car pillar v9 (Autodesk Fusion 360 design; units mm, degrees)
Autodesk Fusion 360 part; units mm, degrees
note: some values were not read from the file. Chosen so that the rebuilt part matches the saved one: which bodies a step acts on; which face or edge a step refers to; the layout of a text. Set by a fixed rule: which sketch regions a step uses.
sketch "Sketch1" plane through (0, 0, 0) normal (0, 1, 0) x (1, 0, 0)
  line L0 (0, 0) -> (75, 0)
  line L1 (75, 0) -> (1014.8, 0)
  line L2 (1014.8, 0) -> (1014.8, -406)
  line L3 (1014.8, -406) -> (913.8, -406)
  arc A0 (75, 0) -> (913.8, -406) centre (913.8, 663.4845) ccw
  line L4 (1014.8, -406) -> (1014.8, -481)
  line L5 (1014.8, -481) -> (913.8, -481)
  arc A1 (0, 0) -> (913.8, -481) centre (913.8, 627.515) ccw
  dimension "d1" = 75
  dimension "d2" = 939.8
  dimension "d3" = 406
  dimension "d4" = 101
  dimension "d5" = 75
  dimension "d6" = 101
  constraint coincident L0.start A1.start
  constraint horizontal L0
  constraint parallel L0 L1
  constraint perpendicular L1 L2
  constraint perpendicular L2 L3
  constraint tangent L3 A0
  constraint perpendicular L3 L4
  constraint perpendicular L4 L5
  constraint tangent L5 A1
  measures "d1" distance of L0.start L0.end
  measures "d2" distance of L0.end L1.end
  measures "d3" distance of L1.end L2.end
  measures "d4" distance of L2.end L3.end
  measures "d5" distance of L2.end L4.end
  measures "d6" distance of L4.end L5.end
extrude "Extrude1" add sketch "Sketch1" along normal blind 76.2 contours L0 L3 A0 L4 L5 A1 makes body 1
sketch "Sketch2" plane through (0, 0, 0) normal (0, -1, 0) x (1, 0, 0)
  line L0 (0, 0) -> (75, 0)
  arc A0 (913.8, 406) -> (75, 0) centre (913.8, -663.4845) ccw
  line L1 (913.8, 406) -> (1014.8, 406)
  line L2 (1014.8, 406) -> (1014.8, 481)
  line L3 (1014.8, 481) -> (913.8, 481)
  arc A1 (913.8, 481) -> (0, 0) centre (913.8, -627.515) ccw
  line L4 (75, 0, -76.2) -> (0, 0, -76.2)
  arc A2 through (913.8, 481, -76.2) (397.4688, 353.4068, -76.2) (0, 0, -76.2)
  line L5 (913.8, 481, -76.2) -> (1014.8, 481, -76.2)
  line L6 (1014.8, 481, -76.2) -> (1014.8, 406, -76.2)
  line L7 (1014.8, 406, -76.2) -> (913.8, 406, -76.2)
  arc A3 through (913.8, 406, -76.2) (447.8543, 299.1638, -76.2) (75, 0, -76.2)
  arc A4 (913.8, 406) -> (75, 0) centre (913.8, -663.4845) ccw
  line L8 (178.7478, 202.2463) -> (217.2163, 148.0376)
  line L9 (317.7078, 307.0863) -> (348.9045, 244.64)
  line L10 (466.2211, 386.6244) -> (489.3869, 318.1827)
  line L11 (629.2604, 443.8592) -> (639.0355, 370.1022)
  line L12 (787.0542, 473.7302) -> (796.8801, 399.5897)
  line L13 (99.0687, 124.162) -> (134.4845, 68.9528)
  line L14 (913.8, 481) -> (913.8, 406)
  constraint coincident A1 L8.start
  constraint coincident A0 L8.end
  constraint coincident A1 L9.start
  constraint coincident A4 L9.end
  constraint coincident A1 L10.start
  constraint coincident A0 L10.end
  constraint coincident A1 L11.start
  constraint coincident A4 L11.end
  constraint coincident A1 L12.start
  constraint coincident A4 L12.end
  constraint parallel L11 L12
  constraint coincident A1 L13.start
  constraint coincident A0 L13.end
  constraint coincident L3.end A1.start
  constraint coincident A0.start L1.start
split "Split1" by curves path "Sketch2" along L8 bodies 1 makes body 2 at (156.5161, 50.8, 182.0074)
split "Split2" by curves path "Sketch2" along L13 bodies 2 makes body 3 at (20.4596, 25.4, 28.7993)
split "Split3" by curves path "Sketch2" along L9 L11 L12 L10 L14 bodies 1 makes body 4 at (301.4758, 50.8, 296.5329) makes body 5 at (333.5896, 50.8, 317.028) makes body 6 at (981.1333, 25.4, 406) makes body 7 at (555.7045, 50.8, 421.567) makes body 8 at (769.3289, 50.8, 471.5453)
fillet "Fillet1" radius 37.5 22 edges at (855.2522, 0, 404.3962) (964.3, 0, 406) (964.3, 76.2, 406) (855.2522, 76.2, 404.3962) (417.7808, 76.2, 284.0186) (281.2137, 76.2, 198.8563) (717.4036, 76.2, 387.8126) (563.2486, 76.2, 346.9168) (104.008, 76.2, 35.1098) (174.7917, 76.2, 109.6027) (174.7917, 0, 109.6027) (174.7917, 76.2, 109.6027) (104.008, 0, 35.1098) (104.008, 76.2, 35.1098) (563.2486, 0, 346.9168) (563.2486, 76.2, 346.9168) (717.4036, 0, 387.8126) (717.4036, 76.2, 387.8126) (281.2137, 0, 198.8563) (281.2137, 76.2, 198.8563) (417.7808, 0, 284.0186) (417.7808, 76.2, 284.0186) on bodies 1 2 3 4 5 6 7 8
shell "Shell2" thickness 3.5 removed faces 1 at (769.3289, 50.8, 471.5453) on bodies 8
shell "Shell3" thickness 3.5 removed faces 1 at (555.7045, 50.8, 421.567) on bodies 7
shell "Shell4" thickness 3.5 removed faces 1 at (333.5896, 50.8, 317.028) on bodies 5
shell "Shell5" thickness 3.5 removed faces 1 at (301.4758, 50.8, 296.5329) on bodies 4
shell "Shell6" thickness 3.5 removed faces 1 at (142.3659, 50.8, 168.5346) on bodies 2
shell "Shell7" thickness 3.5 removed faces 1 at (20.4596, 25.4, 28.7993) on bodies 3
shell "Shell8" thickness 3.5 removed faces 1 at (885.5756, 50.8, 480.6406) on bodies 1
shell "Shell9" thickness 3.5 removed faces 1 at (947.4667, 50.8, 481) on bodies 6
sketch "Sketch3" plane through (1014.8, 0, 0) normal (1, 0, 0) x (0, 1, 0)
  arc A0 (38.7, 406) -> (76.2, 443.5) centre (38.7, 443.5) ccw
  line L0 (76.2, 443.5) -> (76.2, 481)
  line L1 (76.2, 481) -> (0, 481)
  line L2 (0, 481) -> (0, 443.5)
  arc A1 (0, 443.5) -> (37.5, 406) centre (37.5, 443.5) ccw
  line L3 (37.5, 406) -> (38.7, 406)
  line L4 (38.1, 473.1824) -> (38.1, 422.3824)
  circle A2 centre (38.1, 427.3824) radius 5
  circle A3 centre (38.1, 468.1824) radius 5
  dimension "d21" = 38.1
  dimension "d22" = 50.8
  dimension "d23" = 7.8176
  dimension "d24" = 10
  dimension "d25" = 10
  constraint vertical L4
  constraint coincident L4.end A2
  constraint coincident L4.start A3
  measures "d21" distance of L2 L4
  measures "d22" distance of L4.start L4.end
  measures "d23" distance of L1 L4.start
  measures "d24" diameter of A2
  measures "d25" diameter of A3
extrude "Extrude2" cut sketch "Sketch3" against normal blind 10 contours L4 A3 | L4 A3 | L4 A2 | L4 A2 bodies 6
sketch "Sketch4" plane through (917.3, 0, 0) normal (1, 0, 0) x (0, 1, 0)
  arc A0 (38.7, 409.5) -> (72.7, 443.5) centre (38.7, 443.5) ccw
  line L0 (72.7, 443.5) -> (72.7, 481)
  line L1 (72.7, 481) -> (3.5, 481)
  line L2 (3.5, 481) -> (3.5, 443.5)
  arc A1 (3.5, 443.5) -> (37.5, 409.5) centre (37.5, 443.5) ccw
  line L3 (37.5, 409.5) -> (38.7, 409.5)
  line L4 (3.5, 481) -> (72.7, 481)
  line L5 (38.1, 481) -> (38.1, 430.2)
  line L6 (38.1, 481) -> (38.1, 468.3)
  line L7 (38.1, 430.2) -> (58.1, 430.2)
  line L8 (38.1, 430.2) -> (18.1, 430.2)
  circle A2 centre (18.1, 430.2) radius 1.575
  circle A3 centre (58.1, 430.2) radius 1.575
  circle A4 centre (38.1, 468.3) radius 1.575
  line L9 (33.6, 450.6777) -> (42.6, 450.6777) construction
  line L10 (42.6, 450.6777) -> (42.6, 461) construction
  line L11 (42.6, 461) -> (33.6, 461) construction
  line L12 (33.6, 461) -> (33.6, 450.6777) construction
  dimension "d28" = 90
  dimension "d29" = 50.8
  dimension "d30" = 12.7
  dimension "d31" = 20
  dimension "d32" = 20
  dimension "d33" = 3.15
  dimension "d34" = 3.15
  dimension "d35" = 3.15
  dimension "d102" = 15
  dimension "d103" = 20
  dimension "d104" = 9
  dimension "d105" = 30.1
  text T0 "7" font "Arial" height 15 bold align centre top in box 9 x 10.3223 at (33.6, 450.6777) x (1, 0) y (0, 1) spacing 1 by line height
  constraint coincident L1.end L2.start
  constraint coincident L0.end L1.start
  constraint midpoint L4 L5.start
  constraint perpendicular L4 L6
  constraint perpendicular L5 L7
  constraint horizontal L8
  constraint coincident L8.end A2.centre
  constraint coincident L7.end A3.centre
  constraint coincident L6.end A4.centre
  measures "d28" angle of L4 L5
  measures "d29" distance of L5.start L5.end
  measures "d30" distance of L5.start L6.end
  measures "d31" distance of L5.end L7.end
  measures "d32" distance of L5.end L8.end
  measures "d33" diameter of A2
  measures "d34" diameter of A3
  measures "d35" diameter of A4
  measures "d104" distance of L10
  measures "d105" distance of L2 L12
extrude "Extrude11" cut sketch "Sketch4" against normal blind 1.5 text T0 bodies 6
extrude "Extrude3" cut sketch "Sketch4" against normal blind 16 contours L5 L6 A4 | L5 L6 A4 | A2 | A3 bodies 1 6
sketch "Sketch6" plane through (838.6384, 0, 111.1453) normal (0.991332, 0, 0.131382) x (0, 1, 0)
  spline S0 degree 3 poles (38.7, 294.8481) (40.7978, 294.8481) (43.0889, 295.0551) (47.5758, 295.9478) (49.7717, 296.6335) (53.6482, 298.2395) (55.6859, 299.3078) (59.4901, 301.8503) (61.2567, 303.3244) (64.2239, 306.2922) (65.6979, 308.0594) (68.2402, 311.8649) (69.3084, 313.9032) (70.9144, 317.7812) (71.6002, 319.9783) (72.493, 324.4676) (72.7, 326.7598) (72.7, 328.8587) knots 10.072074 10.072074 10.072074 10.072074 10.70142 10.70142 11.330765 11.330765 11.960214 11.960214 12.589663 12.589663 13.219234 13.219234 13.848804 13.848804 14.478468 14.478468 15.108132 15.108132 15.108132 15.108132
  line L0 (72.7, 328.8587) -> (72.7, 366.1536)
  line L1 (72.7, 366.1536) -> (3.5, 366.1536)
  line L2 (3.5, 366.1536) -> (3.5, 328.8587)
  spline S1 degree 3 poles (3.5, 328.8587) (3.5, 326.7598) (3.707, 324.4676) (4.5998, 319.9783) (5.2856, 317.7812) (6.8916, 313.9032) (7.9598, 311.8649) (10.5021, 308.0594) (11.9761, 306.2922) (14.9433, 303.3244) (16.7099, 301.8503) (20.5141, 299.3078) (22.5518, 298.2395) (26.4283, 296.6335) (28.6242, 295.9478) (33.1111, 295.0551) (35.4022, 294.8481) (37.5, 294.8481) knots 5.036017 5.036017 5.036017 5.036017 5.665681 5.665681 6.295345 6.295345 6.924915 6.924915 7.554485 7.554485 8.183935 8.183935 8.813384 8.813384 9.442729 9.442729 10.072074 10.072074 10.072074 10.072074
  line L3 (37.5, 294.8481) -> (38.7, 294.8481)
  line L4 (72.7, 328.5) -> (72.7, 366)
  line L5 (72.7, 366) -> (3.5, 366)
  line L6 (3.5, 366) -> (3.5, 328.5)
  line L7 (37.5, 294.5) -> (38.7, 294.5)
  circle A0 centre (58.1, 315.2) radius 1.575
  arc A1 (3.5, 328.5) -> (37.5, 294.5) centre (37.5, 328.5) ccw
  line L8 (3.5, 366) -> (72.7, 366)
  arc A2 (38.7, 294.5) -> (72.7, 328.5) centre (38.7, 328.5) ccw
  circle A3 centre (38.1, 353.3) radius 1.575
  line L9 (38.1, 315.2) -> (58.1, 315.2)
  circle A4 centre (18.1, 315.2) radius 1.575
  line L10 (38.1, 366) -> (38.1, 353.3)
  line L11 (38.1, 366) -> (38.1, 315.2)
  line L12 (38.1, 315.2) -> (18.1, 315.2)
  line L13 (33.6, 335.6777) -> (42.6, 335.6777) construction
  line L14 (42.6, 335.6777) -> (42.6, 346) construction
  line L15 (42.6, 346) -> (33.6, 346) construction
  line L16 (33.6, 346) -> (33.6, 335.6777) construction
  dimension "d38" = 90
  dimension "d39" = 50.8
  dimension "d40" = 12.7
  dimension "d41" = 20
  dimension "d42" = 20
  dimension "d43" = 3.15
  dimension "d44" = 3.15
  dimension "d45" = 3.15
  dimension "d111" = 15
  dimension "d112" = 20
  text T0 "6" font "Arial" height 15 bold align centre top in box 9 x 10.3223 at (33.6, 335.6777) x (1, 0) y (0, 1) spacing 1 by line height
  constraint coincident L5.end L6.start
  constraint coincident L4.end L5.start
  constraint midpoint L10.start L8
  constraint perpendicular L8 L10
  constraint perpendicular L9 L11
  constraint horizontal L12
  constraint coincident A4.centre L12.end
  constraint coincident A0.centre L9.end
  constraint coincident A3.centre L10.end
  measures "d38" angle of L8 L11
  measures "d39" distance of L9.start L10.start
  measures "d40" distance of A3.centre L10.start
  measures "d41" distance of L9.start A0.centre
  measures "d42" distance of L9.start A4.centre
  measures "d43" diameter of A4
  measures "d44" diameter of A0
  measures "d45" diameter of A3
  measures "d112" distance of L5 L15
extrude "Extrude23" cut sketch "Sketch6" against normal blind 1.5 text T0 bodies 1
sketch "Sketch8" plane through (679.6779, 0, 90.0781) normal (0.991332, 0, 0.131382) x (0, 1, 0)
  spline S0 degree 3 poles (3.5, 321.165) (3.5, 319.0465) (3.708, 316.7327) (4.6052, 312.2003) (5.2945, 309.9818) (6.907, 306.0718) (7.9775, 304.0192) (10.5263, 300.1854) (12.0047, 298.4042) (14.9762, 295.4188) (16.7417, 293.9382) (20.5456, 291.3834) (22.584, 290.3093) (26.4564, 288.6981) (28.6461, 288.011) (33.1215, 287.1163) (35.4071, 286.9086) (37.5, 286.9086) knots 5.053211 5.053211 5.053211 5.053211 5.688762 5.688762 6.324314 6.324314 6.957603 6.957603 7.590893 7.590893 8.221264 8.221264 8.851634 8.851634 9.479515 9.479515 10.107395 10.107395 10.107395 10.107395
  line L0 (37.5, 286.9086) -> (38.7, 286.9086)
  spline S1 degree 3 poles (38.7, 286.9086) (40.7929, 286.9086) (43.0785, 287.1163) (47.5539, 288.011) (49.7436, 288.6981) (53.616, 290.3093) (55.6544, 291.3834) (59.4583, 293.9382) (61.2238, 295.4188) (64.1953, 298.4042) (65.6737, 300.1854) (68.2225, 304.0192) (69.293, 306.0718) (70.9055, 309.9818) (71.5948, 312.2003) (72.492, 316.7327) (72.7, 319.0465) (72.7, 321.165) knots 10.107395 10.107395 10.107395 10.107395 10.735276 10.735276 11.363156 11.363156 11.993527 11.993527 12.623898 12.623898 13.257187 13.257187 13.890477 13.890477 14.526028 14.526028 15.16158 15.16158 15.16158 15.16158
  line L1 (72.7, 321.165) -> (72.7, 357.7826)
  line L2 (72.7, 357.7826) -> (3.5, 357.7826)
  line L3 (3.5, 357.7826) -> (3.5, 321.165)
  circle A0 centre (38.1, 345.3) radius 1.575
  circle A1 centre (18.1, 307.2) radius 1.575
  circle A2 centre (58.1, 307.2) radius 1.575
  line L4 (38.1, 307.2) -> (58.1, 307.2)
  line L5 (38.1, 307.2) -> (18.1, 307.2)
  line L6 (38.1, 358) -> (38.1, 307.2)
  line L7 (3.5, 358) -> (72.7, 358)
  line L8 (33.6, 320.6777) -> (42.6, 320.6777) construction
  line L9 (42.6, 320.6777) -> (42.6, 338) construction
  line L10 (42.6, 338) -> (33.6, 338) construction
  line L11 (33.6, 338) -> (33.6, 320.6777) construction
  dimension "d46" = 90
  dimension "d47" = 50.8
  dimension "d48" = 20
  dimension "d49" = 20
  dimension "d50" = 3.15
  dimension "d51" = 3.15
  dimension "d52" = 3.15
  dimension "d113" = 15
  dimension "d114" = 20
  text T0 "5" font "Arial" height 15 bold align centre top in box 9 x 17.3223 at (33.6, 320.6777) x (1, 0) y (0, 1) spacing 1 by line height
  constraint midpoint L6.start L7
  constraint perpendicular L4 L6
  constraint horizontal L5
  constraint coincident A1.centre L5.end
  constraint coincident A2.centre L4.end
  measures "d46" angle of L6 L7
  measures "d47" distance of L4.start L6.start
  measures "d48" distance of A2.centre L4.start
  measures "d49" distance of A1.centre L4.start
  measures "d50" diameter of A1
  measures "d51" diameter of A2
  measures "d52" diameter of A0
  measures "d114" distance of L7 L10
extrude "Extrude21" cut sketch "Sketch8" against normal blind 1.5 text T0 bodies 8
sketch "Sketch9" plane through (539.0252, 0, 182.4465) normal (0.947212, 0, 0.320608) x (0, 1, 0)
  spline S0 degree 3 poles (3.5, 182.3779) (3.5, 180.2718) (3.7074, 177.9716) (4.6018, 173.4665) (5.2889, 171.2616) (6.8973, 167.3718) (7.9663, 165.3282) (10.511, 161.5123) (11.9866, 159.74) (14.9554, 156.7657) (16.7216, 155.2892) (20.5257, 152.7422) (22.5637, 151.6718) (26.4386, 150.0639) (28.6323, 149.3777) (33.1149, 148.4842) (35.404, 148.277) (37.5, 148.277) knots 5.042332 5.042332 5.042332 5.042332 5.674157 5.674157 6.305983 6.305983 6.93692 6.93692 7.567856 7.567856 8.197644 8.197644 8.827432 8.827432 9.456238 9.456238 10.085044 10.085044 10.085044 10.085044
  line L0 (37.5, 148.277) -> (38.7, 148.277)
  spline S1 degree 3 poles (72.7, 182.3779) (72.7, 180.2718) (72.4926, 177.9716) (71.5982, 173.4665) (70.9111, 171.2616) (69.3027, 167.3718) (68.2337, 165.3282) (65.689, 161.5123) (64.2134, 159.74) (61.2446, 156.7657) (59.4784, 155.2892) (55.6743, 152.7422) (53.6363, 151.6718) (49.7614, 150.0639) (47.5677, 149.3777) (43.0851, 148.4842) (40.796, 148.277) (38.7, 148.277) knots 5.042332 5.042332 5.042332 5.042332 5.674157 5.674157 6.305983 6.305983 6.93692 6.93692 7.567856 7.567856 8.197644 8.197644 8.827432 8.827432 9.456238 9.456238 10.085044 10.085044 10.085044 10.085044
  line L1 (72.7, 182.3779) -> (72.7, 217.0489)
  line L2 (72.7, 217.0489) -> (3.5, 217.0489)
  line L3 (3.5, 217.0489) -> (3.5, 182.3779)
  circle A0 centre (38.1, 204.3) radius 1.575
  circle A1 centre (18.1, 166.2) radius 1.575
  circle A2 centre (58.1, 166.2) radius 1.575
  line L4 (38.1, 166.2) -> (58.1, 166.2)
  line L5 (38.1, 166.2) -> (18.1, 166.2)
  line L6 (38.1, 217) -> (38.1, 166.2)
  line L7 (3.5, 217) -> (72.7, 217)
  line L8 (33.6, 190.6777) -> (42.6, 190.6777) construction
  line L9 (42.6, 190.6777) -> (42.6, 197) construction
  line L10 (42.6, 197) -> (33.6, 197) construction
  line L11 (33.6, 197) -> (33.6, 190.6777) construction
  dimension "d53" = 90
  dimension "d54" = 50.8
  dimension "d55" = 20
  dimension "d56" = 20
  dimension "d57" = 3.15
  dimension "d58" = 3.15
  dimension "d59" = 3.15
  dimension "d115" = 15
  dimension "d116" = 20
  text T0 "4\n" font "Arial" height 15 bold align centre top in box 9 x 6.3223 at (33.6, 190.6777) x (1, 0) y (0, 1) spacing 1 by line height
  constraint midpoint L6.start L7
  constraint perpendicular L4 L6
  constraint horizontal L5
  constraint coincident A1.centre L5.end
  constraint coincident A2.centre L4.end
  measures "d53" angle of L6 L7
  measures "d54" distance of L4.start L6.start
  measures "d55" distance of A2.centre L4.start
  measures "d56" distance of A1.centre L4.start
  measures "d57" diameter of A1
  measures "d58" diameter of A2
  measures "d59" diameter of A0
  measures "d116" distance of L7 L10
extrude "Extrude19" cut sketch "Sketch9" against normal blind 1.5 text T0 bodies 7
sketch "Sketch10" plane through (380.1554, 0, 189.9169) normal (0.894579, 0, 0.446911) x (0, 1, 0)
  spline S0 degree 3 poles (3.5, 100.8886) (3.5, 98.78) (3.7075, 96.477) (4.6025, 91.9663) (5.29, 89.7586) (6.8993, 85.8647) (7.9686, 83.8193) (10.5141, 79.9998) (11.9903, 78.2256) (14.9597, 75.2491) (16.7257, 73.7717) (20.5298, 71.2231) (22.5679, 70.1519) (26.4423, 68.5433) (28.6351, 67.857) (33.1163, 66.9632) (35.4046, 66.7559) (37.5, 66.7559) knots 5.044553 5.044553 5.044553 5.044553 5.677139 5.677139 6.309726 6.309726 6.941143 6.941143 7.57256 7.57256 8.202467 8.202467 8.832374 8.832374 9.460991 9.460991 10.089607 10.089607 10.089607 10.089607
  line L0 (37.5, 66.7559) -> (38.7, 66.7559)
  spline S1 degree 3 poles (38.7, 66.7559) (40.7954, 66.7559) (43.0837, 66.9632) (47.5649, 67.857) (49.7577, 68.5433) (53.6321, 70.1519) (55.6702, 71.2231) (59.4743, 73.7717) (61.2403, 75.2491) (64.2097, 78.2256) (65.6859, 79.9998) (68.2314, 83.8193) (69.3007, 85.8647) (70.91, 89.7586) (71.5975, 91.9663) (72.4925, 96.477) (72.7, 98.78) (72.7, 100.8886) knots 10.089607 10.089607 10.089607 10.089607 10.718224 10.718224 11.34684 11.34684 11.976747 11.976747 12.606654 12.606654 13.238072 13.238072 13.869489 13.869489 14.502075 14.502075 15.134661 15.134661 15.134661 15.134661
  line L1 (72.7, 100.8886) -> (72.7, 133.0871)
  line L2 (72.7, 133.0871) -> (3.5, 133.0871)
  line L3 (3.5, 133.0871) -> (3.5, 100.8886)
  circle A0 centre (38.1, 120.3) radius 1.575
  circle A1 centre (18.1, 82.2) radius 1.575
  circle A2 centre (58.1, 82.2) radius 1.575
  line L4 (38.1, 82.2) -> (58.1, 82.2)
  line L5 (38.1, 82.2) -> (18.1, 82.2)
  line L6 (38.1, 133) -> (38.1, 82.2)
  line L7 (3.5, 133) -> (72.7, 133)
  line L8 (33.6, 100.6777) -> (42.6, 100.6777) construction
  line L9 (42.6, 100.6777) -> (42.6, 113) construction
  line L10 (42.6, 113) -> (33.6, 113) construction
  line L11 (33.6, 113) -> (33.6, 100.6777) construction
  dimension "d60" = 90
  dimension "d61" = 50.8
  dimension "d62" = 20
  dimension "d63" = 20
  dimension "d64" = 3.15
  dimension "d65" = 3.15
  dimension "d66" = 3.15
  dimension "d117" = 15
  dimension "d118" = 20
  text T0 "3\n" font "Arial" height 15 bold align centre top in box 9 x 12.3223 at (33.6, 100.6777) x (1, 0) y (0, 1) spacing 1 by line height
  constraint midpoint L6.start L7
  constraint perpendicular L4 L6
  constraint horizontal L5
  constraint coincident A1.centre L5.end
  constraint coincident A2.centre L4.end
  measures "d60" angle of L6 L7
  measures "d61" distance of L4.start L6.start
  measures "d62" distance of A2.centre L4.start
  measures "d63" distance of A1.centre L4.start
  measures "d64" diameter of A1
  measures "d65" diameter of A2
  measures "d66" diameter of A0
  measures "d118" distance of L7 L10
extrude "Extrude17" cut sketch "Sketch10" against normal blind 1.5 text T0 bodies 5
sketch "Sketch11" plane through (217.1883, 0, 154.1249) normal (0.815523, 0, 0.578725) x (0, 1, 0)
  spline S0 degree 3 poles (3.5, 32.9808) (3.5, 30.8724) (3.7075, 28.5697) (4.6025, 24.0595) (5.2899, 21.8521) (6.8991, 17.9585) (7.9684, 15.9133) (10.5138, 12.0941) (11.99, 10.3201) (14.9593, 7.3438) (16.7253, 5.8665) (20.5294, 3.3181) (22.5675, 2.247) (26.4419, 0.6384) (28.6348, -0.0479) (33.1161, -0.9416) (35.4046, -1.1489) (37.5, -1.1489) knots 5.044348 5.044348 5.044348 5.044348 5.676864 5.676864 6.30938 6.30938 6.940753 6.940753 7.572125 7.572125 8.202021 8.202021 8.831917 8.831917 9.460551 9.460551 10.089185 10.089185 10.089185 10.089185
  line L0 (37.5, -1.1489) -> (38.7, -1.1489)
  spline S1 degree 3 poles (38.7, -1.1489) (40.7954, -1.1489) (43.0839, -0.9416) (47.5652, -0.0479) (49.7581, 0.6384) (53.6325, 2.247) (55.6706, 3.3181) (59.4747, 5.8665) (61.2407, 7.3438) (64.21, 10.3201) (65.6862, 12.0941) (68.2316, 15.9133) (69.3009, 17.9585) (70.9101, 21.8521) (71.5975, 24.0595) (72.4925, 28.5697) (72.7, 30.8724) (72.7, 32.9808) knots 10.089185 10.089185 10.089185 10.089185 10.71782 10.71782 11.346454 11.346454 11.97635 11.97635 12.606246 12.606246 13.237618 13.237618 13.868991 13.868991 14.501507 14.501507 15.134023 15.134023 15.134023 15.134023
  line L1 (72.7, 32.9808) -> (72.7, 61.8636)
  line L2 (72.7, 61.8636) -> (3.5, 61.8636)
  line L3 (3.5, 61.8636) -> (3.5, 32.9808)
  circle A0 centre (38.1, 49.3) radius 1.575
  circle A1 centre (18.1, 11.2) radius 1.575
  circle A2 centre (58.1, 11.2) radius 1.575
  line L4 (38.1, 11.2) -> (58.1, 11.2)
  line L5 (38.1, 11.2) -> (18.1, 11.2)
  line L6 (38.1, 62) -> (38.1, 11.2)
  line L7 (3.5, 62) -> (72.7, 62)
  line L8 (33.6, 30.6777) -> (42.6, 30.6777) construction
  line L9 (42.6, 30.6777) -> (42.6, 42) construction
  line L10 (42.6, 42) -> (33.6, 42) construction
  line L11 (33.6, 42) -> (33.6, 30.6777) construction
  dimension "d67" = 90
  dimension "d68" = 50.8
  dimension "d69" = 20
  dimension "d70" = 20
  dimension "d71" = 3.15
  dimension "d72" = 3.15
  dimension "d73" = 3.15
  dimension "d119" = 15
  dimension "d120" = 20
  text T0 "2\n" font "Arial" height 15 bold align centre top in box 9 x 11.3223 at (33.6, 30.6777) x (1, 0) y (0, 1) spacing 1 by line height
  constraint midpoint L6.start L7
  constraint perpendicular L4 L6
  constraint horizontal L5
  constraint coincident A1.centre L5.end
  constraint coincident A2.centre L4.end
  measures "d67" angle of L6 L7
  measures "d68" distance of L4.start L6.start
  measures "d69" distance of A2.centre L4.start
  measures "d70" distance of A1.centre L4.start
  measures "d71" diameter of A1
  measures "d72" diameter of A2
  measures "d73" diameter of A0
  measures "d120" distance of L7 L10
sketch "Sketch12" plane through (129.5605, 0, 83.1109) normal (0.841704, 0, 0.539939) x (0, 1, 0)
  spline S0 degree 3 poles (3.5, 24.889) (3.5, 22.712) (3.7107, 20.3338) (4.6211, 15.6731) (5.3208, 13.3906) (6.9523, 9.3854) (8.0294, 7.2905) (10.5974, 3.3727) (12.0886, 1.55) (15.0727, -1.4876) (16.8352, -2.9874) (20.638, -5.5785) (22.6783, -6.6695) (26.5385, -8.2963) (28.7105, -8.9874) (33.1519, -9.8882) (35.4214, -10.0976) (37.5, -10.0976) knots 5.104335 5.104335 5.104335 5.104335 5.757428 5.757428 6.41052 6.41052 7.054852 7.054852 7.699183 7.699183 8.33228 8.33228 8.965376 8.965376 9.588969 9.588969 10.212561 10.212561 10.212561 10.212561
  line L0 (37.5, -10.0976) -> (38.7, -10.0976)
  spline S1 degree 3 poles (38.7, -10.0976) (40.7786, -10.0976) (43.0481, -9.8882) (47.4895, -8.9874) (49.6615, -8.2963) (53.5217, -6.6695) (55.562, -5.5785) (59.3648, -2.9874) (61.1273, -1.4876) (64.1114, 1.55) (65.6026, 3.3727) (68.1706, 7.2905) (69.2477, 9.3854) (70.8792, 13.3906) (71.5789, 15.6731) (72.4893, 20.3338) (72.7, 22.712) (72.7, 24.889) knots 10.212561 10.212561 10.212561 10.212561 10.836154 10.836154 11.459746 11.459746 12.092843 12.092843 12.725939 12.725939 13.37027 13.37027 14.014602 14.014602 14.667694 14.667694 15.320787 15.320787 15.320787 15.320787
  line L1 (72.7, 24.889) -> (72.7, 51.924)
  line L2 (72.7, 51.924) -> (3.5, 51.924)
  line L3 (3.5, 51.924) -> (3.5, 24.889)
  circle A0 centre (38.1, 39.3) radius 1.575
  circle A1 centre (18.1, 1.2) radius 1.575
  circle A2 centre (58.1, 1.2) radius 1.575
  line L4 (38.1, 1.2) -> (58.1, 1.2)
  line L5 (38.1, 1.2) -> (18.1, 1.2)
  line L6 (38.1, 52) -> (38.1, 1.2)
  line L7 (3.5, 52) -> (72.7, 52)
  line L8 (33.6, 15.6777) -> (42.6, 15.6777) construction
  line L9 (42.6, 15.6777) -> (42.6, 32) construction
  line L10 (42.6, 32) -> (33.6, 32) construction
  line L11 (33.6, 32) -> (33.6, 15.6777) construction
  dimension "d74" = 90
  dimension "d75" = 50.8
  dimension "d76" = 20
  dimension "d77" = 20
  dimension "d78" = 3.15
  dimension "d79" = 3.15
  dimension "d80" = 3.15
  dimension "d121" = 15
  dimension "d122" = 20
  text T0 "1" font "Arial" height 15 bold align centre top in box 9 x 16.3223 at (33.6, 15.6777) x (1, 0) y (0, 1) spacing 1
  constraint midpoint L6.start L7
  constraint perpendicular L4 L6
  constraint horizontal L5
  constraint coincident A1.centre L5.end
  constraint coincident A2.centre L4.end
  measures "d74" angle of L6 L7
  measures "d75" distance of L4.start L6.start
  measures "d76" distance of A2.centre L4.start
  measures "d77" distance of A1.centre L4.start
  measures "d78" diameter of A1
  measures "d79" diameter of A2
  measures "d80" diameter of A0
  measures "d122" distance of L7 L10
extrude "Extrude13" cut sketch "Sketch12" against normal blind 1.5 text T0 bodies 2
sketch "Sketch13" plane through (0, 0, 3.5) normal (0, 0, 1) x (-1, 0, 0)
  spline S0 degree 3 poles (-30.3146, -3.5) (-33.1455, -3.5) (-36.2433, -3.7391) (-42.3405, -4.7821) (-45.3398, -5.587) (-50.4015, -7.409) (-52.9559, -8.5508) (-57.7905, -11.3054) (-60.0693, -12.9207) (-63.6697, -16.0282) (-65.367, -17.7563) (-68.3369, -21.538) (-69.6069, -23.5937) (-71.3927, -27.3373) (-72.1223, -29.3358) (-73.0805, -33.4467) (-73.3076, -35.5595) (-73.3076, -37.5) knots 5.665376 5.665376 5.665376 5.665376 6.514642 6.514642 7.363909 7.363909 8.128533 8.128533 8.893157 8.893157 9.555324 9.555324 10.217492 10.217492 10.799638 10.799638 11.381784 11.381784 11.381784 11.381784
  line L0 (-73.3076, -37.5) -> (-73.3076, -38.7)
  spline S1 degree 3 poles (-73.3076, -38.7) (-73.3076, -40.6405) (-73.0805, -42.7533) (-72.1223, -46.8642) (-71.3927, -48.8627) (-69.6069, -52.6063) (-68.3369, -54.662) (-65.367, -58.4437) (-63.6697, -60.1718) (-60.0693, -63.2793) (-57.7905, -64.8946) (-52.9559, -67.6492) (-50.4015, -68.791) (-45.3398, -70.613) (-42.3405, -71.4179) (-36.2433, -72.4609) (-33.1455, -72.7) (-30.3146, -72.7) knots 11.381784 11.381784 11.381784 11.381784 11.963931 11.963931 12.546077 12.546077 13.208244 13.208244 13.870412 13.870412 14.635036 14.635036 15.39966 15.39966 16.248926 16.248926 17.098193 17.098193 17.098193 17.098193
  line L1 (-30.3146, -72.7) -> (-2.4134, -72.7)
  line L2 (-2.4134, -72.7) -> (-2.4134, -3.5)
  line L3 (-2.4134, -3.5) -> (-30.3146, -3.5)
  circle A0 centre (-14.9, -38.2) radius 1.575
  circle A1 centre (-53, -18.2) radius 1.575
  circle A2 centre (-53, -58.2) radius 1.575
  line L4 (-53, -38.2) -> (-53, -58.2)
  line L5 (-53, -38.2) -> (-53, -18.2)
  line L6 (-2.2, -38.2) -> (-53, -38.2)
  line L7 (-2.2, -3.6) -> (-2.2, -72.8)
  dimension "d81" = 90
  dimension "d82" = 50.8
  dimension "d83" = 20
  dimension "d84" = 20
  dimension "d85" = 3.15
  dimension "d86" = 3.15
  dimension "d87" = 3.15
  constraint midpoint L6.start L7
  constraint perpendicular L4 L6
  constraint coincident A1.centre L5.end
  constraint coincident A2.centre L4.end
  measures "d81" angle of L6 L7
  measures "d82" distance of L4.start L6.start
  measures "d83" distance of A2.centre L4.start
  measures "d84" distance of A1.centre L4.start
  measures "d85" diameter of A1
  measures "d86" diameter of A2
  measures "d87" diameter of A0
extrude "Extrude4" cut sketch "Sketch13" against normal blind 15 contours A0 L6 | A0 L6 | A1 | A2 bodies 3
extrude "Extrude5" cut sketch "Sketch12" against normal blind 15 contours A0 L6 | A0 L6 | A1 | A2 bodies 2 3
extrude "Extrude6" cut sketch "Sketch11" against normal blind 15 contours A0 L6 | A0 L6 | A1 | A2 bodies 2 4
extrude "Extrude7" cut sketch "Sketch10" against normal blind 15 contours A0 L6 | A0 L6 | A1 | A2 bodies 4 5
extrude "Extrude8" cut sketch "Sketch9" against normal blind 15 contours A0 L6 | A0 L6 | A1 | A2 bodies 7 5
extrude "Extrude9" cut sketch "Sketch8" against normal blind 15 contours A0 L6 | A0 L6 | A1 | A2 bodies 7 8
extrude "Extrude10" cut sketch "Sketch6" against normal blind 15 contours A0 | A3 L10 L11 | A3 L10 L11 | A4 bodies 1 8
extrude "Extrude12" cut 1 faces at (915.8, 38.6201, 455.9352) along direction (-1, 0, 0) blind 9 from surface at 4 on bodies 6 bodies 1
extrude "Extrude14" cut 1 faces at (114.4581, 40.4363, 103.8758) along direction (-0.841704, 0, -0.539939) blind 1.5 from surface at 4 on bodies 2 bodies 3
extrude "Extrude15" cut sketch "Sketch11" against normal blind 1.5 text T0 bodies 4
extrude "Extrude16" cut 1 faces at (202.1218, 37.6106, 172.7642) along direction (-0.815523, 0, -0.578725) blind 1.5 from surface at 4 on bodies 4 bodies 2
extrude "Extrude18" cut 1 faces at (333.1797, 39.0082, 280.5915) along direction (-0.894579, 0, -0.446911) blind 1.5 from surface at 4 on bodies 5 bodies 4
extrude "Extrude20" cut 1 faces at (477.1839, 40.6563, 360.4738) along direction (-0.947212, 0, -0.320608) blind 1.5 from surface at 4 on bodies 7 bodies 5
extrude "Extrude22" cut 1 faces at (634.9036, 35.1106, 416.5019) along direction (-0.991332, 0, -0.131382) blind 1.5 from surface at 4 on bodies 8 bodies 7
extrude "Extrude24" cut 1 faces at (793.2156, 35.3066, 442.4627) along direction (-0.991332, 0, -0.131382) blind 1.5 from surface at 4 on bodies 1 bodies 8
named bodies: "part7", "part2", "part1", "part3", "part4", "part8", "part5", "part6"
